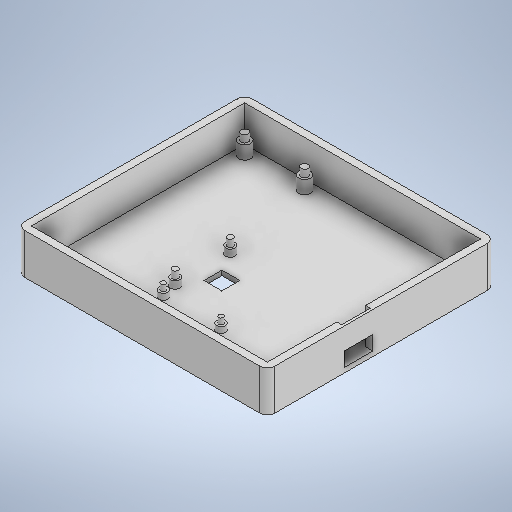
# Autodesk Inventor part: Enclosure
Saved by Autodesk Inventor 2025.2 (Build 292293000, 293)
## iProperties
Created: 2025-04-29
Part Number: Enclosure
Material: Generic
Document SubType Name: Modeling
Designer: mathe
Density: 1 g/cm^3
Appearance: Default
Author: mathe
Autodesk Inventor part; units mm, degrees
ref_plane "YZ Plane" through (0, 0, 0) normal (1, 0, 0) x (0, 1, 0)
ref_plane "XZ Plane" through (0, 0, 0) normal (0, 1, 0) x (-1, 0, 0)
ref_plane "XY Plane" through (0, 0, 0) normal (0, 0, 1) x (1, 0, 0)
sketch "Sketch1" plane through (0, 0, 0) normal (0, 1, 0) x (-1, 0, 0)
  circle A0 centre (0, 0) radius 1.25
  line L0 (0, 0) -> (-58, 0) construction
  line L1 (0, 0) -> (58, 0) construction
  circle A1 centre (-58, 0) radius 1.25
  line L2 (0, 0) -> (0, -23) construction
  line L3 (0, 0) -> (23, 0) construction
  line L4 (0, -23) -> (-58, -23) construction
  line L5 (-58, -23) -> (-58, 0) construction
  circle A2 centre (-58, -23) radius 1.25
  circle A3 centre (0, -23) radius 1.25
  line L6 (-61.5, 3.5) -> (3.5, 3.5)
  line L7 (3.5, 3.5) -> (3.5, -26.5)
  line L8 (3.5, -26.5) -> (-61.5, -26.5)
  line L9 (-61.5, -26.5) -> (-61.5, 3.5)
  line L10 (-61.5, 3.5) -> (3.5, -26.5) construction
  line L11 (3.5, 3.5) -> (-61.5, -26.5) construction
  circle A4 centre (0, 0) radius 2
  circle A5 centre (0, -23) radius 2
  circle A6 centre (-58, -23) radius 2
  circle A7 centre (-58, 0) radius 2
  line L12 (3.5, 3.5) -> (-61.5, 3.5)
  line L13 (-61.5, 3.5) -> (-61.5, 4)
  line L14 (-61.5, 4) -> (3.5, 4)
  line L15 (3.5, 4) -> (3.5, 3.5)
  line L16 (3.5, 4) -> (-28.25, 4)
  line L17 (-28.25, 4) -> (-28.25, 23.05)
  line L18 (-28.25, 23.05) -> (3.5, 23.05)
  line L19 (3.5, 23.05) -> (3.5, 4)
  line L20 (-58, -11.5) -> (0, -11.5) construction
  line L21 (-29, -23) -> (-29, 0) construction
  line L22 (3.5, 23.05) -> (-1.58, 23.05)
  line L23 (-1.58, 23.05) -> (-1.58, 20.51) construction
  line L24 (-1.58, 20.51) -> (3.5, 20.51) construction
  line L25 (3.5, 20.51) -> (3.5, 23.05)
  circle A8 centre (-1.58, 20.51) radius 1.016
  line L26 (3.5, 4) -> (-1.58, 4)
  line L27 (-1.58, 4) -> (-1.58, 6.54) construction
  line L28 (-1.58, 6.54) -> (3.5, 6.54) construction
  line L29 (3.5, 6.54) -> (3.5, 4)
  line L30 (-28.25, 4) -> (-25.71, 4)
  line L31 (-25.71, 4) -> (-25.71, 6.54) construction
  line L32 (-25.71, 6.54) -> (-28.25, 6.54) construction
  line L33 (-28.25, 6.54) -> (-28.25, 4)
  line L34 (-28.25, 23.05) -> (-25.71, 23.05)
  line L35 (-25.71, 23.05) -> (-25.71, 20.51) construction
  line L36 (-25.71, 20.51) -> (-28.25, 20.51) construction
  line L37 (-28.25, 20.51) -> (-28.25, 23.05)
  circle A9 centre (-25.71, 20.51) radius 1.016
  circle A10 centre (-25.71, 6.54) radius 1.016
  circle A11 centre (-1.58, 6.54) radius 1.016
  circle A12 centre (-1.58, 20.51) radius 1.905
  circle A13 centre (-1.58, 6.54) radius 1.905
  circle A14 centre (-25.71, 6.54) radius 1.905
  circle A15 centre (-25.71, 20.51) radius 1.905
  line L38 (3.5, -26.5) -> (-61.5, -26.5)
  line L39 (-61.5, -26.5) -> (-61.5, -27)
  line L40 (-61.5, -27) -> (3.5, -27)
  line L41 (3.5, -27) -> (3.5, -26.5)
  line L42 (3.5, -27) -> (-58.65, -27)
  line L43 (-58.65, -27) -> (-58.65, -65)
  line L44 (-58.65, -65) -> (3.5, -65)
  line L45 (3.5, -65) -> (3.5, -27)
  line L46 (3.5, 23.05) -> (4, 23.05)
  line L47 (4, 23.05) -> (4, -65)
  line L48 (4, -65) -> (3.5, -65)
  line L49 (3.5, -65) -> (3.5, 23.05)
  line L50 (4, -65) -> (36, -65)
  line L51 (36, -65) -> (36, 22)
  line L52 (36, 22) -> (4, 22)
  line L53 (4, 22) -> (4, -65)
  line L54 (36, -21.5) -> (4, -21.5) construction
  line L55 (20, -65) -> (20, 22) construction
  line L56 (7.5, -61.5) -> (32.5, -61.5) construction
  line L57 (32.5, -61.5) -> (32.5, 18.5) construction
  line L58 (32.5, 18.5) -> (7.5, 18.5) construction
  line L59 (7.5, 18.5) -> (7.5, -61.5) construction
  line L60 (7.5, -61.5) -> (32.5, 18.5) construction
  line L61 (32.5, -61.5) -> (7.5, 18.5) construction
  circle A16 centre (32.5, 18.5) radius 1.5
  circle A17 centre (7.5, 18.5) radius 1.5
  circle A18 centre (7.5, -61.5) radius 1.5
  circle A19 centre (32.5, -61.5) radius 1.5
  circle A20 centre (32.5, 18.5) radius 2.5
  circle A21 centre (7.5, 18.5) radius 2.5
  circle A22 centre (32.5, -61.5) radius 2.5
  circle A23 centre (7.5, -61.5) radius 2.5
  line L62 (4, 23.05) -> (-28.25, 23.05)
  line L63 (-28.25, 23.05) -> (-28.25, 23.55)
  line L64 (-28.25, 23.55) -> (4, 23.55)
  line L65 (4, 23.55) -> (4, 23.05)
  line L66 (36, 22) -> (36.5, 22)
  line L67 (36.5, 22) -> (36.5, -65)
  line L68 (36.5, -65) -> (36, -65)
  line L69 (36, -65) -> (36, 22)
  line L70 (36.5, -65) -> (-58.65, -65)
  line L71 (-58.65, -65) -> (-58.65, -65.5)
  line L72 (-58.65, -65.5) -> (36.5, -65.5)
  line L73 (36.5, -65.5) -> (36.5, -65)
  line L74 (-61.5, 4) -> (-62, 4)
  line L75 (-62, 4) -> (-62, -27)
  line L76 (-62, -27) -> (-61.5, -27)
  line L77 (-61.5, -27) -> (-61.5, 4)
  line L78 (-62, 23.55) -> (36.5, 23.55)
  line L79 (36.5, 23.55) -> (36.5, -65.5)
  line L80 (36.5, -65.5) -> (-62, -65.5)
  line L81 (-62, -65.5) -> (-62, 23.55)
  line L82 (-65, 26.55) -> (39.5, 26.55)
  line L83 (39.5, 26.55) -> (39.5, -68.5)
  line L84 (39.5, -68.5) -> (-65, -68.5)
  line L85 (-65, -68.5) -> (-65, 26.55)
  line L86 (3.5, 3.5) -> (-8, 3.5)
  line L87 (-8, 3.5) -> (-8, -26.5) construction
  line L88 (-8, -26.5) -> (3.5, -26.5)
  line L89 (3.5, -26.5) -> (3.5, 3.5)
  line L90 (-11.75, -7.75) -> (-4.25, -7.75)
  line L91 (-4.25, -7.75) -> (-4.25, -15.25)
  line L92 (-4.25, -15.25) -> (-11.75, -15.25)
  line L93 (-11.75, -15.25) -> (-11.75, -7.75)
  line L94 (-11.75, -7.75) -> (-4.25, -15.25) construction
  line L95 (-4.25, -7.75) -> (-11.75, -15.25) construction
  point P0 (-29, -11.5)
  point P1 (20, -21.5)
  point P2 (-8, -11.5)
  dimension "d0" = 2.5
  dimension "d1" = 58
  dimension "d2" = 180
  dimension "d3" = 2.5
  dimension "d4" = 23
  dimension "d5" = 270
  dimension "d6" = 90
  dimension "d7" = 2.5
  dimension "d8" = 2.5
  dimension "d9" = 65
  dimension "d10" = 30
  dimension "d11" = 4
  dimension "d12" = 4
  dimension "d13" = 4
  dimension "d14" = 4
  dimension "d15" = 0.5
  dimension "d16" = 31.75
  dimension "d17" = 19.05
  dimension "d18" = 5.08
  dimension "d19" = 2.54
  dimension "d20" = 2.032
  dimension "d21" = 5.08
  dimension "d22" = 2.54
  dimension "d23" = 2.54
  dimension "d24" = 2.54
  dimension "d25" = 2.54
  dimension "d26" = 2.54
  dimension "d27" = 2.032
  dimension "d28" = 2.032
  dimension "d29" = 2.032
  dimension "d30" = 3.81
  dimension "d31" = 3.81
  dimension "d32" = 3.81
  dimension "d33" = 3.81
  dimension "d34" = 0.5
  dimension "d35" = 62.15
  dimension "d36" = 38
  dimension "d37" = 0.5
  dimension "d38" = 32
  dimension "d39" = 87
  dimension "d40" = 25
  dimension "d41" = 80
  dimension "d42" = 3
  dimension "d43" = 3
  dimension "d44" = 3
  dimension "d45" = 3
  dimension "d46" = 5
  dimension "d47" = 5
  dimension "d48" = 5
  dimension "d49" = 5
  dimension "d50" = 0.5
  dimension "d51" = 0.5
  dimension "d52" = 0.5
  dimension "d53" = 0.5
  dimension "d56" = 3
  dimension "d59" = 11.5
  dimension "d60" = 7.5
  dimension "d61" = 7.5
  constraints: 192 end point, 40 parallel, 24 centre point, 24 coincident, 22 horizontal, 21 perpendicular, 18 midpoint, 9 collinear, 2 equal length, 1 point on line, 1 vertical, 3 other
  measures "d0" diameter of A0
  measures "d1" distance of L0.start L0.end
  measures "d2" angle of L0 L1
  measures "d3" diameter of A1
  measures "d4" distance of L0.start L2.end
  measures "d6" angle of L2 L4
  measures "d7" diameter of A2
  measures "d8" diameter of A3
  measures "d9" distance of L7.end L8.end
  measures "d10" distance of L6.end L7.end
  measures "d11" diameter of A4
  measures "d12" diameter of A5
  measures "d13" diameter of A6
  measures "d14" diameter of A7
  measures "d15" distance of L12.end L13.end
  measures "d16" distance of L17.end L18.end
  measures "d17" distance of L16.end L17.end
  measures "d18" distance of L23.end L24.end
  measures "d19" distance of L22.end L23.end
  measures "d20" diameter of A8
  measures "d21" distance of L27.end L28.end
  measures "d22" distance of L26.end L27.end
  measures "d23" distance of L32.end L31.end
  measures "d24" distance of L31.end L30.end
  measures "d25" distance of L35.end L36.end
  measures "d26" distance of L34.end L35.end
  measures "d27" diameter of A9
  measures "d28" diameter of A10
  measures "d29" diameter of A11
  measures "d30" diameter of A12
  measures "d31" diameter of A13
  measures "d32" diameter of A14
  measures "d33" diameter of A15
  measures "d34" distance of L39.end L38.end
  measures "d35" distance of L44.end L43.end
  measures "d36" distance of L43.end L42.end
  measures "d37" distance of L47.end L48.end
  measures "d38" distance of L52.end L51.end
  measures "d39" distance of L51.end L50.end
  measures "d40" distance of L58.end L57.end
  measures "d41" distance of L57.end L56.end
  measures "d42" diameter of A16
  measures "d43" diameter of A17
  measures "d44" diameter of A18
  measures "d45" diameter of A19
  measures "d46" diameter of A20
  measures "d47" diameter of A21
  measures "d48" diameter of A22
  measures "d49" diameter of A23
  measures "d50" distance of L62.end L63.end
  measures "d51" distance of L67.end L68.end
  measures "d52" distance of L71.end L70.end
  measures "d53" distance of L76.end L75.end
  measures "d56" distance between parallel lines of L81 L85
  measures "d59" distance of L88.end L87.end
  measures "d60" distance of L91.end L92.end
  measures "d61" distance of L90.end L91.end
extrude "Extrusion1" add sketch "Sketch1" against normal blind 2 contours A0 | A1 | A2 | A3 | L13 L14 L15 L6 | L6 L7 L8 L9 | L9 L39 L76 L75 L74 L13 | L8 L41 L40 L39 | L74 L81 L78 L63 L17 L14 | L15 L19 L46 L47 L48 L45 L41 L7 | L40 L43 L71 L80 L81 L76 | L17 L18 L19 L14 | L40 L45 L44 L43 | L44 L48 L50 L68 L73 L72 L71 | L64 L65 L46 L18 L63 | L78 L79 L66 L52 L47 L65 | L47 L52 L51 L50 | L51 L66 L67 L68 | A4 | A5 | A6 | A7 | A8 | A9 | A10 | A11 | A12 | A13 | A14 | A15 | A16 | A17 | A18 | A19 | A20 | A21 | A22 | A23 | L82 L83 L84 L85 | L90 L91 L92 L93
extrude "Extrusion2" add sketch "Sketch1" along normal blind 15 contours L82 L83 L84 L85
extrude "Extrusion3" cut sketch "Sketch1" against normal up to surface (2 mm away) contours L90 L91 L92 L93
extrude "Extrusion4" add sketch "Sketch1" along normal blind 5.5 contours A20 | A21 | A22 | A23
extrude "Extrusion5" add sketch "Sketch1" along normal blind 8.5 contours A16 | A17 | A18 | A19
extrude "Extrusion6" add sketch "Sketch1" along normal blind 3 contours A4 | A5 | A6 | A7
extrude "Extrusion7" add sketch "Sketch1" along normal blind 6 contours A0 | A1 | A2 | A3
extrude "Extrusion8" add sketch "Sketch1" along normal blind 2.5 contours A12 | A13 | A14 | A15
extrude "Extrusion9" add sketch "Sketch1" along normal blind 5 contours A8 | A9 | A10 | A11
sketch "Sketch2" plane through (65, -2, 26.55) normal (1, 0, 0) x (0, 0, -1)
  line L0 (28.55, 5) -> (24.55, 5) projected
  line L1 (51.55, 5) -> (47.55, 5) projected
  line L2 (24.55, 5) -> (51.55, 5) construction
  line L3 (44.05, 8) -> (32.05, 8)
  line L4 (32.05, 8) -> (32.05, 2)
  line L5 (32.05, 2) -> (44.05, 2)
  line L6 (44.05, 2) -> (44.05, 8)
  line L7 (44.05, 8) -> (32.05, 2) construction
  line L8 (32.05, 8) -> (44.05, 2) construction
  line L9 (44.05, 8) -> (56.05, 8) construction
  point P0 (26.55, 2)
  point P1 (38.05, 5)
  dimension "d76" = 12
  dimension "d77" = 180
  constraints: 16 end point, 3 midpoint, 3 parallel, 2 horizontal, 1 collinear, 1 perpendicular
  measures "d76" distance of L3.start L3.end
  measures "d77" angle of L3 L9
extrude "Extrusion10" cut sketch "Sketch2" against normal up to surface (3 mm away)
sketch "Sketch3" plane through (0, 15, 0) normal (0, 1, 0) x (1, 0, 0)
  circle A0 centre (25.71, -6.54) radius 1.905 projected
  circle A1 centre (1.58, -6.54) radius 1.905 projected
  circle A2 centre (25.71, -20.51) radius 1.905 projected
  circle A3 centre (1.58, -20.51) radius 1.905 projected
  circle A4 centre (58, 23) radius 2 projected
  circle A5 centre (0, 23) radius 2 projected
  circle A6 centre (58, 0) radius 2 projected
  circle A7 centre (0, 0) radius 2 projected
  circle A8 centre (-32.5, 61.5) radius 2.5 projected
  circle A9 centre (-32.5, -18.5) radius 2.5 projected
  circle A10 centre (-7.5, 61.5) radius 2.5 projected
  circle A11 centre (-7.5, -18.5) radius 2.5 projected
  line L0 (11.75, 15.25) -> (11.75, 7.75) projected
  line L1 (11.75, 7.75) -> (4.25, 7.75) projected
  line L2 (4.25, 7.75) -> (4.25, 15.25) projected
  line L3 (4.25, 15.25) -> (11.75, 15.25) projected
  line L4 (62, 65.5) -> (-36.5, 65.5) projected
  line L5 (-36.5, 65.5) -> (-36.5, -23.55) projected
  line L6 (-36.5, -23.55) -> (62, -23.55) projected
  line L7 (62, -23.55) -> (62, 5.5) projected
  line L8 (65, 5.5) -> (62, 5.5) projected
  line L9 (65, 17.5) -> (65, 5.5) projected
  line L10 (65, 17.5) -> (62, 17.5) projected
  line L11 (62, 17.5) -> (62, 65.5) projected
  line L12 (62, 5.5) -> (64, 5.5)
  line L13 (64, 5.5) -> (64, 17.5)
  line L14 (64, 17.5) -> (62, 17.5)
  line L15 (62, 17.5) -> (62, 5.5)
  dimension "d80" = 2
  constraints: 8 end point, 2 parallel, 1 horizontal, 1 perpendicular, 1 point on line
  measures "d80" distance of L14.end L13.end
extrude "Extrusion11" cut sketch "Sketch3" against normal up to surface (9 mm away) contours L10 L13 L8 L15
fillet "Fillet1" radius 3.175 4 edges at (65, 6.5, 26.55) (65, 6.5, -68.5) (-39.5, 6.5, -68.5) (-39.5, 6.5, 26.55)
body "Solid1"
